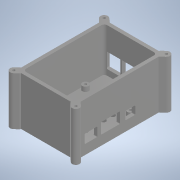
# Autodesk Inventor part: Case RevB
Saved by Autodesk Inventor 2021 (Build 250183000, 183)
## iProperties
Created: 2021-07-24
Part Number: Case RevB
Material: ABS Plastic
Document SubType Name: Modeling
Designer: cmzgt
Density: 0.1 g/cm^3
Appearance: Smooth - White
Author: cmzgt
Autodesk Inventor part; units mm, degrees
ref_plane "YZ Plane" through (0, 0, 0) normal (1, 0, 0) x (0, 1, 0)
ref_plane "XZ Plane" through (0, 0, 0) normal (0, 1, 0) x (-1, 0, 0)
ref_plane "XY Plane" through (0, 0, 0) normal (0, 0, 1) x (1, 0, 0)
sketch "Sketch1" plane through (0, 0, 0) normal (0, 1, 0) x (-1, 0, 0)
  line L0 (-32.55, -48.25) -> (32.55, -48.25)
  line L1 (32.55, -48.25) -> (32.55, 48.25)
  line L2 (32.55, 48.25) -> (-32.55, 48.25)
  line L3 (-32.55, 48.25) -> (-32.55, -48.25)
  line L4 (-32.55, -48.25) -> (32.55, 48.25) construction
  line L5 (32.55, -48.25) -> (-32.55, 48.25) construction
  point P0 (0, 0)
  dimension "d0" = 65.1
  dimension "d1" = 96.5
  constraints: 12 end point, 2 midpoint, 2 parallel, 1 horizontal, 1 perpendicular
  measures "d0" distance of L2.end L1.end
  measures "d1" distance of L0.end L1.end
extrude "Extrusion1" add sketch "Sketch1" along normal blind 5.08
sketch "Sketch2" plane through (0, 5.08, 0) normal (0, 1, 0) x (1, 0, 0)
  line L0 (28.75, 44.45) -> (-28.75, 44.45)
  line L1 (-28.75, 44.45) -> (-28.75, -44.45)
  line L2 (-28.75, -44.45) -> (28.75, -44.45)
  line L3 (28.75, -44.45) -> (28.75, 44.45)
  line L4 (28.75, 44.45) -> (-28.75, -44.45) construction
  line L5 (-28.75, 44.45) -> (28.75, -44.45) construction
  line L6 (-32.55, 48.25) -> (-32.55, -48.25) projected
  line L7 (-32.55, -48.25) -> (32.55, -48.25) projected
  line L8 (32.55, 48.25) -> (-32.55, 48.25) projected
  line L9 (32.55, -48.25) -> (32.55, 48.25) projected
  line L10 (24.95, -40.65) -> (32.55, -48.25) construction
  line L11 (23.0931, -44.45) -> (29.7216, -51.0784)
  line L12 (35.3784, -45.4216) -> (28.75, -38.7931)
  arc A0 (29.7216, -51.0784) -> (35.3784, -45.4216) centre (32.55, -48.25) ccw
  circle A1 centre (32.55, -48.25) radius 1.375
  point P0 (0, 0)
  dimension "d4" = 3.8
  dimension "d5" = 3.8
  dimension "d22" = 8
  dimension "d23" = 2.75
  constraints: 20 end point, 4 parallel, 3 midpoint, 2 centre point, 2 point on circle, 2 point on line, 2 tangent, 1 coincident, 1 horizontal, 1 perpendicular
  measures "d4" distance between parallel lines of L6 L1
  measures "d5" distance between parallel lines of L7 L2
  measures "d22" diameter of A0
  measures "d23" diameter of A1
extrude "Extrusion2" add sketch "Sketch2" along normal blind 48 contours L0 L1 L2 L11 L7 L6 L8 L9 L12 L3 | L12 L9 A1 L7 L11 L2 L3 | L9 L7 A1 picked at (32.448, -47.3448)
sketch "Sketch3" plane through (0, 5.08, 0) normal (0, 1, 0) x (1, 0, 0)
  line L0 (28.75, -44.45) -> (-28.75, -44.45) construction
  line L1 (0, -44.45) -> (0, 44.45) construction
  line L2 (28.75, 44.45) -> (-28.75, 44.45) construction
  circle A0 centre (-24.5, -38.45) radius 3.5
  circle A1 centre (-24.5, -38.45) radius 1.375
  line L3 (28.75, 44.45) -> (28.75, -44.45) construction
  line L4 (28.75, 0) -> (-28.75, 0) construction
  line L5 (-28.75, -44.45) -> (-28.75, 44.45) construction
  circle A2 centre (-24.5, 19.55) radius 3.5
  circle A3 centre (-24.5, 19.55) radius 1.375
  circle A4 centre (24.5, -38.45) radius 3.5
  circle A5 centre (24.5, -38.45) radius 1.375
  circle A6 centre (24.5, 19.55) radius 3.5
  circle A7 centre (24.5, 19.55) radius 1.375
  point P0 (0, 0)
  dimension "d8" = 7
  dimension "d9" = 2.75
  dimension "d10" = 6
  dimension "d11" = 24.5
  dimension "d14" = 58
  constraints: 8 centre point, 4 coincident, 4 end point, 4 midpoint, 4 symmetric about line, 1 vertical, 8 other
  measures "d8" diameter of A0
  measures "d9" diameter of A1
  measures "d10" distance from line of L0 A0.centre
  measures "d11" distance from line of L1 A1.centre
  measures "d14" distance of A0.centre A2.centre
extrude "Extrusion3" add sketch "Sketch3" along normal blind 5
sketch "Sketch4" plane through (0, 0, 0) normal (0, -1, 0) x (1, 0, 0)
  line L0 (31.0438, 46.9342) -> (34.0562, 49.5658) construction
  line L1 (32.55, 48.25) -> (32.55, -48.25) projected
  line L2 (32.55, 42.9386) -> (36.6878, 46.5534)
  line L3 (31.4245, 52.5782) -> (28.4122, 49.9466)
  arc A0 (28.4122, 49.9466) -> (27.2664, 48.25) centre (31.0438, 46.9342) ccw
  arc A1 (36.6878, 46.5534) -> (31.4245, 52.5782) centre (34.0562, 49.5658) ccw
  line L4 (-32.55, 48.25) -> (32.55, 48.25) projected
  line L5 (27.2664, 48.25) -> (32.55, 48.25)
  line L6 (32.55, 48.25) -> (32.55, 42.9386)
  circle A2 centre (34.0562, 49.5658) radius 1.375
  line L7 (0, 48.25) -> (0, -48.25) construction
  line L8 (32.55, -48.25) -> (-32.55, -48.25) construction
  line L9 (32.55, 0) -> (-33.3, 0) construction
  line L10 (32.55, -48.25) -> (32.55, 48.25)
  line L11 (32.55, -42.9386) -> (36.6878, -46.5534)
  line L12 (31.4245, -52.5782) -> (28.4122, -49.9466)
  arc A3 (27.2664, -48.25) -> (28.4122, -49.9466) centre (31.0438, -46.9342) ccw
  arc A4 (31.4245, -52.5782) -> (36.6878, -46.5534) centre (34.0562, -49.5658) ccw
  line L13 (-32.55, -48.25) -> (32.55, -48.25)
  circle A5 centre (34.0562, -49.5658) radius 1.375
  line L14 (-32.55, 48.25) -> (-32.55, -48.25)
  line L15 (-32.55, 42.9386) -> (-36.6878, 46.5534)
  line L16 (-31.4245, 52.5782) -> (-28.4122, 49.9466)
  arc A6 (-27.2664, 48.25) -> (-28.4122, 49.9466) centre (-31.0438, 46.9342) ccw
  arc A7 (-31.4245, 52.5782) -> (-36.6878, 46.5534) centre (-34.0562, 49.5658) ccw
  line L17 (-27.2664, 48.25) -> (-32.55, 48.25)
  circle A8 centre (-34.0562, 49.5658) radius 1.375
  arc A9 (-36.6878, -46.5534) -> (-31.4245, -52.5782) centre (-34.0562, -49.5658) ccw
  line L18 (-32.55, -42.9386) -> (-36.6878, -46.5534)
  line L19 (-31.4245, -52.5782) -> (-28.4122, -49.9466)
  arc A10 (-28.4122, -49.9466) -> (-27.2664, -48.25) centre (-31.0438, -46.9342) ccw
  circle A11 centre (-34.0562, -49.5658) radius 1.375
  line L20 (-27.2664, -48.25) -> (-32.55, -48.25)
  line L21 (-32.55, -48.25) -> (-32.55, 48.25)
  point P0 (0, 0)
  point P1 (-32.55, -42.9386)
  point P2 (32.55, -48.25)
  dimension "d24" = 2
  dimension "d25" = 8
  dimension "d26" = 131.141
  dimension "d27" = 2.75
  constraints: 40 end point, 30 symmetric about line, 16 point on circle, 12 centre point, 6 point on line, 4 coincident, 4 midpoint, 4 tangent, 1 collinear, 1 horizontal, 1 parallel, 9 other
  measures "d24" distance of L1.start L0.end
  measures "d25" diameter of A1
  measures "d26" angle of L1 L2
  measures "d27" diameter of A2
extrude "Extrusion4" add sketch "Sketch4" against normal up to surface (53.08 mm away) contours L4 A0 L3 A1 L2 L1 | L11 A4 L12 A3 L13 L1 | L4 L14 L15 A7 L16 A6 | A10 L19 A9 L18 L14 L13
fillet "Fillet2" radius 3 4 edges at (28.75, 29.08, -44.45) (-28.75, 29.08, -44.45) (-28.75, 29.08, 44.45) (28.75, 29.08, 44.45)
sketch "Sketch5" plane through (0, 5.08, 0) normal (0, 1, 0) x (1, 0, 0)
  line L0 (15, 0) -> (-15, 0) construction
  line L1 (15, 2.5) -> (-15, 2.5)
  line L2 (-15, -2.5) -> (15, -2.5)
  arc A0 (15, -2.5) -> (15, 2.5) centre (15, 0) ccw
  arc A1 (-15, 2.5) -> (-15, -2.5) centre (-15, 0) ccw
  line L3 (-25.75, -44.45) -> (25.75, -44.45) construction
  line L4 (0, -44.45) -> (0, 44.45) construction
  line L5 (-25.75, 44.45) -> (25.75, 44.45) construction
  arc A2 (-15, 12.5) -> (-15, 7.5) centre (-15, 10) ccw
  line L6 (15, 12.5) -> (-15, 12.5)
  line L7 (-15, 7.5) -> (15, 7.5)
  arc A3 (15, 7.5) -> (15, 12.5) centre (15, 10) ccw
  arc A4 (-15, 22.5) -> (-15, 17.5) centre (-15, 20) ccw
  line L8 (15, 22.5) -> (-15, 22.5)
  line L9 (-15, 17.5) -> (15, 17.5)
  arc A5 (15, 17.5) -> (15, 22.5) centre (15, 20) ccw
  arc A6 (-15, 32.5) -> (-15, 27.5) centre (-15, 30) ccw
  line L10 (15, 32.5) -> (-15, 32.5)
  line L11 (-15, 27.5) -> (15, 27.5)
  arc A7 (15, 27.5) -> (15, 32.5) centre (15, 30) ccw
  arc A8 (-15, -7.5) -> (-15, -12.5) centre (-15, -10) ccw
  line L12 (-15, -12.5) -> (15, -12.5)
  line L13 (15, -7.5) -> (-15, -7.5)
  arc A9 (15, -12.5) -> (15, -7.5) centre (15, -10) ccw
  arc A10 (-15, -17.5) -> (-15, -22.5) centre (-15, -20) ccw
  line L14 (-15, -22.5) -> (15, -22.5)
  line L15 (15, -17.5) -> (-15, -17.5)
  arc A11 (15, -22.5) -> (15, -17.5) centre (15, -20) ccw
  arc A12 (-15, -27.5) -> (-15, -32.5) centre (-15, -30) ccw
  line L16 (-15, -32.5) -> (15, -32.5)
  line L17 (15, -27.5) -> (-15, -27.5)
  arc A13 (15, -32.5) -> (15, -27.5) centre (15, -30) ccw
  point P0 (0, 0)
  dimension "d31" = 15
  dimension "d32" = 5
  dimension "d35" = 10
  dimension "d42" = 10
  constraints: 34 end point, 28 point on circle, 14 centre point, 4 tangent, 3 midpoint, 2 vertical, 1 horizontal, 1 parallel, 60 other
  measures "d31" distance of point (0, 0) L0.end
  measures "d32" diameter of A1
  measures "d35" distance of L0.end A2.centre
  measures "d42" distance of L0.end A8.centre
extrude "Extrusion5" cut sketch "Sketch5" against normal up to surface (5.08 mm away)
sketch "Sketch9" plane through (27.2664, 0, -48.25) normal (0, 0, -1) x (-1, 0, 0)
  line L0 (6.2664, 10.08) -> (-0.7336, 10.08) projected
  line L1 (1.3914, 10.08) -> (4.1414, 10.08) projected
  line L2 (1.3914, 10.08) -> (4.1414, 10.08) construction
  line L3 (2.7664, 10.08) -> (-0.7336, 10.08) construction
  line L4 (6.2664, 10.08) -> (-0.7336, 10.08) projected
  line L5 (0, 53.08) -> (0, 0) projected
  line L6 (-0.7336, 10.08) -> (0, 13.5023) construction
  line L7 (17.725, 11.35) -> (1.475, 11.35)
  line L8 (1.475, 11.35) -> (1.475, 25.6)
  line L9 (1.475, 25.6) -> (17.725, 25.6)
  line L10 (17.725, 25.6) -> (17.725, 11.35)
  line L11 (9.6, 25.6) -> (9.6, 11.35) construction
  line L12 (20.5, 11.35) -> (36.5, 11.35)
  line L13 (36.5, 11.35) -> (36.5, 27.85)
  line L14 (36.5, 27.85) -> (20.5, 27.85)
  line L15 (20.5, 27.85) -> (20.5, 11.35)
  line L16 (28.5, 27.85) -> (28.5, 11.35) construction
  line L17 (54.5, 27.85) -> (38.5, 27.85)
  line L18 (54.5, 11.35) -> (54.5, 27.85)
  line L19 (38.5, 11.35) -> (54.5, 11.35)
  line L20 (38.5, 27.85) -> (38.5, 11.35)
  point P0 (27.2664, 0)
  point P1 (46.5, 27.85)
  point P2 (46.5, 11.35)
  dimension "d58" = 3.5
  dimension "d60" = 3.5
  dimension "d63" = 16.25
  dimension "d64" = 14.25
  dimension "d65" = 1.27
  dimension "d66" = 9.6
  dimension "d69" = 16
  dimension "d70" = 16.5
  dimension "d71" = 1.27
  dimension "d72" = 28.5
  dimension "d75" = 18
  constraints: 32 end point, 5 midpoint, 4 parallel, 3 horizontal, 2 perpendicular, 1 collinear, 1 point on line, 10 other
  measures "d58" distance of L3.start L0.end
  measures "d60" distance of L0.end L6.end
  measures "d63" distance of L8.end L9.end
  measures "d64" distance of L7.end L8.end
  measures "d65" distance between parallel lines of L0 L7
  measures "d66" distance between parallel lines of L5 L11
  measures "d69" distance of L14.end L13.end
  measures "d70" distance of L12.end L13.end
  measures "d71" distance between parallel lines of L4 L12
  measures "d72" distance between parallel lines of L5 L16
  measures "d75" distance of L13.end L17.start
extrude "Extrusion7" cut sketch "Sketch9" against normal up to surface (3.8 mm away)
sketch "Sketch11" plane through (32.55, 0, 42.9386) normal (1, 0, 0) x (0, 0, -1)
  line L0 (4.5402, 20.48) -> (18.5209, 20.48)
  line L1 (18.5209, 20.48) -> (18.5209, 10.48)
  line L2 (18.5209, 10.48) -> (4.5402, 10.48)
  line L3 (4.5402, 10.48) -> (4.5402, 20.48)
  line L4 (22.4305, 22.48) -> (43.4305, 22.48)
  line L5 (43.4305, 22.48) -> (43.4305, 10.48)
  line L6 (43.4305, 10.48) -> (22.4305, 10.48)
  line L7 (22.4305, 10.48) -> (22.4305, 22.48)
  line L8 (25.4305, 16.69) -> (25.4305, 14.2116)
  line L9 (40.4305, 14.2116) -> (40.4305, 16.69)
  line L10 (15.5209, 13.09) -> (15.5209, 12.8971)
  line L11 (7.5402, 12.8971) -> (7.5402, 13.09)
  line L12 (82.9128, 10.28) -> (3.9886, 10.28)
  line L13 (49.0305, 19.78) -> (60.0305, 19.78)
  line L14 (60.0305, 19.78) -> (60.0305, 10.78)
  line L15 (60.0305, 10.78) -> (49.0305, 10.78)
  line L16 (49.0305, 10.78) -> (49.0305, 19.78)
  line L17 (51.0305, 17.41) -> (51.0305, 11.41)
  line L18 (58.0305, 11.41) -> (58.0305, 17.41)
  point P0 (42.9386, 0)
extrude "Extrusion8" cut sketch "Sketch11" against normal up to surface (3.8 mm away)
fillet "Fillet4" radius 1 12 edges at (30.65, 22.48, -0.492) (30.65, 22.48, 20.508) (30.65, 10.48, 20.508) (30.65, 10.48, -0.492) (30.65, 19.78, -6.092) (30.65, 10.78, -6.092) (30.65, 10.78, -17.092) (30.65, 19.78, -17.092) (30.65, 20.48, 24.4177) (30.65, 20.48, 38.3984) (30.65, 10.48, 38.3984) (30.65, 10.48, 24.4177)
body "Solid1"
